Autodesk Fusion 360 part; units mm, degrees
note: some values were not read from the file. Set by a fixed rule: which sketch regions a step uses.
(part 30 of 59)
  spline S54 degree 5 poles (20.9575, -7.61) (20.9576, -7.61) (20.9577, -7.6102) (20.958, -7.6104) (20.9583, -7.6107) (20.9589, -7.6112) (20.9595, -7.6118) (20.9602, -7.6125) (20.961, -7.6132) (20.9619, -7.614) (20.9629, -7.6149) (20.9639, -7.6159) (20.9651, -7.6169) (20.9663, -7.618) (20.9675, -7.6192) (20.9689, -7.6204) (20.9704, -7.6217) (20.9719, -7.623) (20.9735, -7.6245) (20.9752, -7.626) (20.9769, -7.6275) (20.9787, -7.6291) (20.9806, -7.6308) (20.9826, -7.6325) (20.9847, -7.6343) (20.9868, -7.6361) (20.989, -7.638) (20.9912, -7.6399) (20.9936, -7.6419) (20.996, -7.644) (20.9984, -7.6461) (21.001, -7.6482) (21.0036, -7.6504) (21.0063, -7.6527) (21.009, -7.655) (21.0119, -7.6573) (21.0148, -7.6597) (21.0177, -7.6622) (21.0207, -7.6647) (21.0238, -7.6672) (21.027, -7.6698) (21.0302, -7.6724) (21.0335, -7.6751) (21.0368, -7.6778) (21.0403, -7.6806) (21.0437, -7.6834) (21.0473, -7.6862) (21.0509, -7.6891) (21.0546, -7.692) (21.0583, -7.695) (21.0621, -7.698) (21.066, -7.701) (21.0699, -7.7041) (21.0739, -7.7072) (21.0779, -7.7103) (21.082, -7.7135) (21.0862, -7.7167) (21.0904, -7.72) (21.0947, -7.7233) (21.099, -7.7266) (21.1034, -7.73) (21.1079, -7.7333) (21.1124, -7.7368) (21.117, -7.7402) (21.1216, -7.7437) (21.1263, -7.7472) (21.1311, -7.7508) (21.1359, -7.7544) (21.1408, -7.758) (21.1457, -7.7616) (21.1507, -7.7653) (21.1557, -7.769) (21.1608, -7.7727) (21.166, -7.7765) (21.1712, -7.7802) (21.1764, -7.7841) (21.1818, -7.7879) (21.1871, -7.7918) (21.1926, -7.7956) (21.1981, -7.7996) (21.2036, -7.8035) (21.2092, -7.8075) (21.2148, -7.8115) (21.2205, -7.8155) (21.2263, -7.8195) (21.2321, -7.8236) (21.238, -7.8277) (21.2439, -7.8318) (21.2498, -7.8359) (21.2559, -7.8401) (21.2619, -7.8442) (21.2681, -7.8484) (21.2742, -7.8527) (21.2805, -7.8569) (21.2867, -7.8612) (21.2931, -7.8655) (21.2995, -7.8698) (21.3059, -7.8741) (21.3124, -7.8784) (21.3189, -7.8828) (21.3255, -7.8872) (21.3321, -7.8916) (21.3388, -7.896) (21.3455, -7.9004) (21.3523, -7.9049) (21.3592, -7.9094) (21.3661, -7.9139) (21.373, -7.9184) (21.38, -7.9229) (21.387, -7.9274) (21.3941, -7.932) (21.4012, -7.9366) (21.4084, -7.9412) (21.4156, -7.9458) (21.4229, -7.9504) (21.4302, -7.955) (21.4376, -7.9597) (21.445, -7.9644) (21.4525, -7.969) (21.46, -7.9737) (21.4676, -7.9784) (21.4752, -7.9832) (21.4828, -7.9879) (21.4905, -7.9927) (21.4983, -7.9974) (21.5061, -8.0022) (21.5139, -8.007) (21.5218, -8.0118) (21.5297, -8.0166) (21.5377, -8.0214) (21.5458, -8.0263) (21.5538, -8.0311) (21.5619, -8.036) (21.5701, -8.0409) (21.5783, -8.0457) (21.5866, -8.0506) (21.5949, -8.0555) (21.6032, -8.0605) (21.6116, -8.0654) (21.6201, -8.0703) (21.6285, -8.0753) (21.6371, -8.0802) (21.6456, -8.0852) (21.6542, -8.0902) (21.6629, -8.0951) (21.6716, -8.1001) (21.6803, -8.1051) (21.6891, -8.1101) (21.698, -8.1152) (21.7068, -8.1202) (21.7158, -8.1252) (21.7247, -8.1303) (21.7337, -8.1353) (21.7428, -8.1404) (21.7519, -8.1454) (21.761, -8.1505) (21.7702, -8.1556) (21.7794, -8.1607) (21.7887, -8.1658) (21.798, -8.1709) (21.8073, -8.176) (21.8167, -8.1811) (21.8261, -8.1862) (21.8356, -8.1913) (21.8451, -8.1965) (21.8547, -8.2016) (21.8643, -8.2067) (21.8739, -8.2119) (21.8836, -8.217) (21.8933, -8.2222) (21.9031, -8.2274) (21.9129, -8.2325) (21.9228, -8.2377) (21.9326, -8.2429) (21.9426, -8.248) (21.9525, -8.2532) (21.9625, -8.2584) (21.9726, -8.2636) (21.9827, -8.2688) (21.9928, -8.274) (22.003, -8.2792) (22.0132, -8.2844) (22.0235, -8.2896) (22.0337, -8.2948) (22.0441, -8.3) (22.0544, -8.3052) (22.0649, -8.3105) (22.0753, -8.3157) (22.0858, -8.3209) (22.0963, -8.3261) (22.1069, -8.3313) (22.1175, -8.3366) (22.1281, -8.3418) (22.1388, -8.347) (22.1496, -8.3523) (22.1603, -8.3575) (22.1711, -8.3627) (22.182, -8.368) (22.1928, -8.3732) (22.2038, -8.3784) (22.2147, -8.3837) (22.2257, -8.3889) (22.2367, -8.3942) (22.2478, -8.3994) (22.2589, -8.4046) (22.2701, -8.4099) (22.2812, -8.4151) (22.2925, -8.4204) (22.3037, -8.4256) (22.315, -8.4308) (22.3264, -8.4361) (22.3377, -8.4413) (22.3491, -8.4466) (22.3606, -8.4518) (22.3721, -8.457) (22.3836, -8.4623) (22.3951, -8.4675) (22.4067, -8.4727) (22.4184, -8.478) (22.43, -8.4832) (22.4417, -8.4884) (22.4535, -8.4937) (22.4653, -8.4989) (22.4771, -8.5041) (22.4889, -8.5093) (22.5008, -8.5145) (22.5127, -8.5198) (22.5247, -8.525) (22.5367, -8.5302) (22.5487, -8.5354) (22.5608, -8.5406) (22.5729, -8.5458) (22.585, -8.551) (22.5972, -8.5562) (22.6094, -8.5614) (22.6217, -8.5666) (22.6339, -8.5718) (22.6462, -8.577) (22.6586, -8.5822) (22.671, -8.5873) (22.6834, -8.5925) (22.6934, -8.5967) (22.7009, -8.5998) (22.7059, -8.6018) (22.7084, -8.6029) knots 0 0 0 0 0 0 0.00416667 0.00833333 0.0125 0.01666667 0.02083333 0.025 0.02916667 0.03333333 0.0375 0.04166667 0.04583333 0.05 0.05416667 0.05833333 0.0625 0.06666667 0.07083333 0.075 0.07916667 0.08333333 0.0875 0.09166667 0.09583333 0.1 0.10416667 0.10833333 0.1125 0.11666667 0.12083333 0.125 0.12916667 0.13333333 0.1375 0.14166667 0.14583333 0.15 0.15416667 0.15833333 0.1625 0.16666667 0.17083333 0.175 0.17916667 0.18333333 0.1875 0.19166667 0.19583333 0.2 0.20416667 0.20833333 0.2125 0.21666667 0.22083333 0.225 0.22916667 0.23333333 0.2375 0.24166667 0.24583333 0.25 0.25416667 0.25833333 0.2625 0.26666667 0.27083333 0.275 0.27916667 0.28333333 0.2875 0.29166667 0.29583333 0.3 0.30416667 0.30833333 0.3125 0.31666667 0.32083333 0.325 0.32916667 0.33333333 0.3375 0.34166667 0.34583333 0.35 0.35416667 0.35833333 0.3625 0.36666667 0.37083333 0.375 0.37916667 0.38333333 0.3875 0.39166667 0.39583333 0.4 0.40416667 0.40833333 0.4125 0.41666667 0.42083333 0.425 0.42916667 0.43333333 0.4375 0.44166667 0.44583333 0.45 0.45416667 0.45833333 0.4625 0.46666667 0.47083333 0.475 0.47916667 0.48333333 0.4875 0.49166667 0.49583333 0.5 0.50416667 0.50833333 0.5125 0.51666667 0.52083333 0.525 0.52916667 0.53333333 0.5375 0.54166667 0.54583333 0.55 0.55416667 0.55833333 0.5625 0.56666667 0.57083333 0.575 0.57916667 0.58333333 0.5875 0.59166667 0.59583333 0.6 0.60416667 0.60833333 0.6125 0.61666667 0.62083333 0.625 0.62916667 0.63333333 0.6375 0.64166667 0.64583333 0.65 0.65416667 0.65833333 0.6625 0.66666667 0.67083333 0.675 0.67916667 0.68333333 0.6875 0.69166667 0.69583333 0.7 0.70416667 0.70833333 0.7125 0.71666667 0.72083333 0.725 0.72916667 0.73333333 0.7375 0.74166667 0.74583333 0.75 0.75416667 0.75833333 0.7625 0.76666667 0.77083333 0.775 0.77916667 0.78333333 0.7875 0.79166667 0.79583333 0.8 0.80416667 0.80833333 0.8125 0.81666667 0.82083333 0.825 0.82916667 0.83333333 0.8375 0.84166667 0.84583333 0.85 0.85416667 0.85833333 0.8625 0.86666667 0.87083333 0.875 0.87916667 0.88333333 0.8875 0.89166667 0.89583333 0.9 0.90416667 0.90833333 0.9125 0.91666667 0.92083333 0.925 0.92916667 0.93333333 0.9375 0.94166667 0.94583333 0.95 0.95416667 0.95833333 0.9625 0.96666667 0.97083333 0.975 0.97916667 0.98333333 0.9875 0.99166667 0.99583333 1 1 1 1 1 1
  arc A63 (22.7084, -8.6029) -> (23.3609, -7.8781) centre (0, 12.5) ccw
  spline S55 degree 5 poles (23.3609, -7.8781) (23.3596, -7.8757) (23.3571, -7.871) (23.3532, -7.8639) (23.348, -7.8544) (23.3416, -7.8426) (23.3351, -7.8308) (23.3287, -7.819) (23.3222, -7.8073) (23.3158, -7.7957) (23.3094, -7.784) (23.3029, -7.7724) (23.2965, -7.7609) (23.29, -7.7493) (23.2836, -7.7379) (23.2771, -7.7264) (23.2707, -7.715) (23.2643, -7.7036) (23.2578, -7.6922) (23.2514, -7.6809) (23.245, -7.6697) (23.2385, -7.6584) (23.2321, -7.6472) (23.2257, -7.636) (23.2193, -7.6249) (23.2128, -7.6138) (23.2064, -7.6028) (23.2, -7.5917) (23.1936, -7.5808) (23.1872, -7.5698) (23.1807, -7.5589) (23.1743, -7.548) (23.1679, -7.5372) (23.1615, -7.5264) (23.1551, -7.5156) (23.1487, -7.5049) (23.1423, -7.4942) (23.136, -7.4836) (23.1296, -7.473) (23.1232, -7.4624) (23.1168, -7.4518) (23.1104, -7.4413) (23.1041, -7.4309) (23.0977, -7.4205) (23.0914, -7.4101) (23.085, -7.3997) (23.0786, -7.3894) (23.0723, -7.3791) (23.066, -7.3689) (23.0596, -7.3587) (23.0533, -7.3486) (23.047, -7.3384) (23.0406, -7.3284) (23.0343, -7.3183) (23.028, -7.3083) (23.0217, -7.2984) (23.0154, -7.2884) (23.0091, -7.2785) (23.0029, -7.2687) (22.9966, -7.2589) (22.9903, -7.2491) (22.984, -7.2394) (22.9778, -7.2297) (22.9715, -7.22) (22.9653, -7.2104) (22.9591, -7.2009) (22.9528, -7.1913) (22.9466, -7.1818) (22.9404, -7.1724) (22.9342, -7.163) (22.928, -7.1536) (22.9218, -7.1443) (22.9156, -7.135) (22.9095, -7.1257) (22.9033, -7.1165) (22.8971, -7.1073) (22.891, -7.0982) (22.8849, -7.0891) (22.8787, -7.0801) (22.8726, -7.0711) (22.8665, -7.0621) (22.8604, -7.0532) (22.8543, -7.0443) (22.8483, -7.0354) (22.8422, -7.0266) (22.8361, -7.0179) (22.8301, -7.0091) (22.8241, -7.0005) (22.818, -6.9918) (22.812, -6.9832) (22.806, -6.9747) (22.8, -6.9662) (22.7941, -6.9577) (22.7881, -6.9493) (22.7822, -6.9409) (22.7762, -6.9325) (22.7703, -6.9242) (22.7644, -6.916) (22.7585, -6.9078) (22.7526, -6.8996) (22.7467, -6.8914) (22.7408, -6.8834) (22.735, -6.8753) (22.7292, -6.8673) (22.7233, -6.8593) (22.7175, -6.8514) (22.7118, -6.8436) (22.706, -6.8357) (22.7002, -6.8279) (22.6945, -6.8202) (22.6887, -6.8125) (22.683, -6.8048) (22.6773, -6.7972) (22.6716, -6.7897) (22.666, -6.7821) (22.6603, -6.7747) (22.6547, -6.7672) (22.6491, -6.7598) (22.6435, -6.7525) (22.6379, -6.7452) (22.6323, -6.7379) (22.6268, -6.7307) (22.6212, -6.7236) (22.6157, -6.7165) (22.6102, -6.7094) (22.6048, -6.7024) (22.5993, -6.6954) (22.5939, -6.6884) (22.5884, -6.6815) (22.583, -6.6747) (22.5777, -6.6679) (22.5723, -6.6611) (22.567, -6.6544) (22.5617, -6.6478) (22.5564, -6.6412) (22.5511, -6.6346) (22.5458, -6.6281) (22.5406, -6.6216) (22.5354, -6.6152) (22.5302, -6.6088) (22.525, -6.6025) (22.5199, -6.5962) (22.5148, -6.59) (22.5097, -6.5838) (22.5046, -6.5776) (22.4996, -6.5715) (22.4945, -6.5655) (22.4895, -6.5595) (22.4846, -6.5536) (22.4796, -6.5477) (22.4747, -6.5418) (22.4698, -6.536) (22.4649, -6.5303) (22.4601, -6.5246) (22.4553, -6.5189) (22.4505, -6.5133) (22.4457, -6.5077) (22.441, -6.5022) (22.4363, -6.4968) (22.4316, -6.4914) (22.427, -6.486) (22.4223, -6.4807) (22.4177, -6.4755) (22.4132, -6.4703) (22.4087, -6.4651) (22.4042, -6.46) (22.3997, -6.455) (22.3953, -6.45) (22.3909, -6.4451) (22.3865, -6.4402) (22.3821, -6.4353) (22.3778, -6.4306) (22.3736, -6.4258) (22.3693, -6.4211) (22.3651, -6.4165) (22.3609, -6.4119) (22.3568, -6.4074) (22.3527, -6.403) (22.3486, -6.3986) (22.3446, -6.3942) (22.3406, -6.3899) (22.3367, -6.3856) (22.3328, -6.3814) (22.3289, -6.3773) (22.325, -6.3732) (22.3212, -6.3692) (22.3175, -6.3652) (22.3138, -6.3613) (22.3101, -6.3574) (22.3065, -6.3536) (22.3029, -6.3499) (22.2993, -6.3462) (22.2958, -6.3426) (22.2923, -6.339) (22.2889, -6.3355) (22.2855, -6.332) (22.2822, -6.3286) (22.2789, -6.3252) (22.2757, -6.322) (22.2725, -6.3187) (22.2693, -6.3156) (22.2662, -6.3124) (22.2632, -6.3094) (22.2602, -6.3064) (22.2572, -6.3035) (22.2543, -6.3006) (22.2515, -6.2978) (22.2487, -6.2951) (22.2459, -6.2924) (22.2433, -6.2897) (22.2406, -6.2872) (22.238, -6.2847) (22.2355, -6.2823) (22.2331, -6.2799) (22.2307, -6.2776) (22.2283, -6.2753) (22.226, -6.2732) (22.2238, -6.271) (22.2216, -6.269) (22.2195, -6.267) (22.2175, -6.2651) (22.2155, -6.2632) (22.2136, -6.2615) (22.2117, -6.2597) (22.2099, -6.2581) (22.2082, -6.2565) (22.2066, -6.255) (22.205, -6.2536) (22.2035, -6.2522) (22.202, -6.2509) (22.2007, -6.2497) (22.1994, -6.2485) (22.1982, -6.2474) (22.197, -6.2464) (22.196, -6.2455) (22.195, -6.2446) (22.1941, -6.2438) (22.1933, -6.2431) (22.1925, -6.2424) (22.1919, -6.2419) (22.1913, -6.2414) (22.1909, -6.241) (22.1907, -6.2408) (22.1905, -6.2407) (22.1904, -6.2406) knots -1 -1 -1 -1 -1 -1 -0.99583333 -0.99166667 -0.9875 -0.98333333 -0.97916667 -0.975 -0.97083333 -0.96666667 -0.9625 -0.95833333 -0.95416667 -0.95 -0.94583333 -0.94166667 -0.9375 -0.93333333 -0.92916667 -0.925 -0.92083333 -0.91666667 -0.9125 -0.90833333 -0.90416667 -0.9 -0.89583333 -0.89166667 -0.8875 -0.88333333 -0.87916667 -0.875 -0.87083333 -0.86666667 -0.8625 -0.85833333 -0.85416667 -0.85 -0.84583333 -0.84166667 -0.8375 -0.83333333 -0.82916667 -0.825 -0.82083333 -0.81666667 -0.8125 -0.80833333 -0.80416667 -0.8 -0.79583333 -0.79166667 -0.7875 -0.78333333 -0.77916667 -0.775 -0.77083333 -0.76666667 -0.7625 -0.75833333 -0.75416667 -0.75 -0.74583333 -0.74166667 -0.7375 -0.73333333 -0.72916667 -0.725 -0.72083333 -0.71666667 -0.7125 -0.70833333 -0.70416667 -0.7 -0.69583333 -0.69166667 -0.6875 -0.68333333 -0.67916667 -0.675 -0.67083333 -0.66666667 -0.6625 -0.65833333 -0.65416667 -0.65 -0.64583333 -0.64166667 -0.6375 -0.63333333 -0.62916667 -0.625 -0.62083333 -0.61666667 -0.6125 -0.60833333 -0.60416667 -0.6 -0.59583333 -0.59166667 -0.5875 -0.58333333 -0.57916667 -0.575 -0.57083333 -0.56666667 -0.5625 -0.55833333 -0.55416667 -0.55 -0.54583333 -0.54166667 -0.5375 -0.53333333 -0.52916667 -0.525 -0.52083333 -0.51666667 -0.5125 -0.50833333 -0.50416667 -0.5 -0.49583333 -0.49166667 -0.4875 -0.48333333 -0.47916667 -0.475 -0.47083333 -0.46666667 -0.4625 -0.45833333 -0.45416667 -0.45 -0.44583333 -0.44166667 -0.4375 -0.43333333 -0.42916667 -0.425 -0.42083333 -0.41666667 -0.4125 -0.40833333 -0.40416667 -0.4 -0.39583333 -0.39166667 -0.3875 -0.38333333 -0.37916667 -0.375 -0.37083333 -0.36666667 -0.3625 -0.35833333 -0.35416667 -0.35 -0.34583333 -0.34166667 -0.3375 -0.33333333 -0.32916667 -0.325 -0.32083333 -0.31666667 -0.3125 -0.30833333 -0.30416667 -0.3 -0.29583333 -0.29166667 -0.2875 -0.28333333 -0.27916667 -0.275 -0.27083333 -0.26666667 -0.2625 -0.25833333 -0.25416667 -0.25 -0.24583333 -0.24166667 -0.2375 -0.23333333 -0.22916667 -0.225 -0.22083333 -0.21666667 -0.2125 -0.20833333 -0.20416667 -0.2 -0.19583333 -0.19166667 -0.1875 -0.18333333 -0.17916667 -0.175 -0.17083333 -0.16666667 -0.1625 -0.15833333 -0.15416667 -0.15 -0.14583333 -0.14166667 -0.1375 -0.13333333 -0.12916667 -0.125 -0.12083333 -0.11666667 -0.1125 -0.10833333 -0.10416667 -0.1 -0.09583333 -0.09166667 -0.0875 -0.08333333 -0.07916667 -0.075 -0.07083333 -0.06666667 -0.0625 -0.05833333 -0.05416667 -0.05 -0.04583333 -0.04166667 -0.0375 -0.03333333 -0.02916667 -0.025 -0.02083333 -0.01666667 -0.0125 -0.00833333 -0.00416667 0 0 0 0 0 0
  line L111 (22.1904, -6.2406) -> (22.1898, -6.2401)
  line L112 (22.1898, -6.2401) -> (21.9649, -6.0501)
  arc A64 (21.9649, -6.0501) -> (22.7115, -5.1281) centre (0, 12.5) ccw
  line L113 (22.7115, -5.1281) -> (22.9441, -5.3086)
  line L114 (22.9441, -5.3086) -> (22.9448, -5.3091)
  spline S56 degree 5 poles (22.9448, -5.3091) (22.9448, -5.3092) (22.945, -5.3093) (22.9453, -5.3095) (22.9457, -5.3098) (22.9463, -5.3103) (22.9469, -5.3108) (22.9477, -5.3114) (22.9486, -5.312) (22.9496, -5.3127) (22.9506, -5.3135) (22.9518, -5.3144) (22.953, -5.3153) (22.9543, -5.3162) (22.9557, -5.3172) (22.9572, -5.3183) (22.9588, -5.3195) (22.9604, -5.3207) (22.9622, -5.3219) (22.964, -5.3232) (22.9659, -5.3246) (22.9679, -5.326) (22.9699, -5.3274) (22.9721, -5.3289) (22.9743, -5.3305) (22.9766, -5.3321) (22.979, -5.3337) (22.9814, -5.3354) (22.984, -5.3372) (22.9866, -5.3389) (22.9893, -5.3408) (22.992, -5.3427) (22.9948, -5.3446) (22.9978, -5.3465) (23.0007, -5.3485) (23.0038, -5.3506) (23.0069, -5.3527) (23.0101, -5.3548) (23.0134, -5.357) (23.0167, -5.3592) (23.0201, -5.3614) (23.0236, -5.3637) (23.0271, -5.366) (23.0308, -5.3683) (23.0344, -5.3707) (23.0382, -5.3731) (23.042, -5.3756) (23.0459, -5.3781) (23.0499, -5.3806) (23.0539, -5.3831) (23.058, -5.3857) (23.0621, -5.3883) (23.0664, -5.391) (23.0706, -5.3937) (23.075, -5.3964) (23.0794, -5.3991) (23.0839, -5.4019) (23.0884, -5.4047) (23.093, -5.4075) (23.0977, -5.4103) (23.1024, -5.4132) (23.1072, -5.4161) (23.1121, -5.4191) (23.117, -5.422) (23.122, -5.425) (23.127, -5.428) (23.1321, -5.431) (23.1373, -5.4341) (23.1425, -5.4372) (23.1478, -5.4403) (23.1531, -5.4434) (23.1585, -5.4466) (23.164, -5.4497) (23.1695, -5.4529) (23.1751, -5.4562) (23.1807, -5.4594) (23.1864, -5.4627) (23.1921, -5.4659) (23.1979, -5.4692) (23.2038, -5.4726) (23.2097, -5.4759) (23.2157, -5.4793) (23.2217, -5.4826) (23.2278, -5.486) (23.234, -5.4895) (23.2402, -5.4929) (23.2464, -5.4963) (23.2527, -5.4998) (23.2591, -5.5033) (23.2655, -5.5068) (23.272, -5.5103) (23.2785, -5.5139) (23.2851, -5.5174) (23.2918, -5.521) (23.2984, -5.5246) (23.3052, -5.5282) (23.312, -5.5318) (23.3188, -5.5354) (23.3257, -5.539) (23.3327, -5.5427) (23.3397, -5.5464) (23.3468, -5.5501) (23.3539, -5.5538) (23.361, -5.5575) (23.3683, -5.5612) (23.3755, -5.5649) (23.3828, -5.5687) (23.3902, -5.5724) (23.3976, -5.5762) (23.4051, -5.58) (23.4126, -5.5838) (23.4202, -5.5876) (23.4278, -5.5914) (23.4355, -5.5952) (23.4432, -5.5991) (23.451, -5.6029) (23.4588, -5.6068) (23.4666, -5.6106) (23.4746, -5.6145) (23.4825, -5.6184) (23.4905, -5.6223) (23.4986, -5.6262) (23.5067, -5.6301) (23.5149, -5.634) (23.5231, -5.6379) (23.5313, -5.6419) (23.5396, -5.6458) (23.548, -5.6498) (23.5564, -5.6537) (23.5648, -5.6577) (23.5733, -5.6617) (23.5818, -5.6657) (23.5904, -5.6696) (23.5991, -5.6736) (23.6077, -5.6776) (23.6165, -5.6816) (23.6252, -5.6857) (23.634, -5.6897) (23.6429, -5.6937) (23.6518, -5.6977) (23.6607, -5.7018) (23.6697, -5.7058) (23.6788, -5.7098) (23.6879, -5.7139) (23.697, -5.7179) (23.7062, -5.722) (23.7154, -5.726) (23.7247, -5.7301) (23.734, -5.7342) (23.7433, -5.7383) (23.7527, -5.7423) (23.7622, -5.7464) (23.7716, -5.7505) (23.7812, -5.7546) (23.7907, -5.7587) (23.8004, -5.7627) (23.81, -5.7668) (23.8197, -5.7709) (23.8295, -5.775) (23.8393, -5.7791) (23.8491, -5.7832) (23.859, -5.7873) (23.8689, -5.7914) (23.8788, -5.7955) (23.8888, -5.7996) (23.8989, -5.8038) (23.909, -5.8079) (23.9191, -5.812) (23.9292, -5.8161) (23.9395, -5.8202) (23.9497, -5.8243) (23.96, -5.8284) (23.9703, -5.8325) (23.9807, -5.8366) (23.9911, -5.8408) (24.0016, -5.8449) (24.0121, -5.849) (24.0226, -5.8531) (24.0332, -5.8572) (24.0438, -5.8613) (24.0545, -5.8654) (24.0652, -5.8695) (24.0759, -5.8736) (24.0867, -5.8777) (24.0975, -5.8818) (24.1084, -5.8859) (24.1193, -5.89) (24.1302, -5.8941) (24.1412, -5.8982) (24.1522, -5.9023) (24.1633, -5.9064) (24.1744, -5.9105) (24.1855, -5.9146) (24.1967, -5.9187) (24.2079, -5.9228) (24.2191, -5.9269) (24.2304, -5.9309) (24.2417, -5.935) (24.2531, -5.9391) (24.2645, -5.9431) (24.276, -5.9472) (24.2874, -5.9513) (24.299, -5.9553) (24.3105, -5.9594) (24.3221, -5.9634) (24.3337, -5.9675) (24.3454, -5.9715) (24.3571, -5.9756) (24.3689, -5.9796) (24.3806, -5.9836) (24.3925, -5.9877) (24.4043, -5.9917) (24.4162, -5.9957) (24.4281, -5.9997) (24.4401, -6.0037) (24.4521, -6.0077) (24.4642, -6.0117) (24.4762, -6.0157) (24.4884, -6.0197) (24.5005, -6.0237) (24.5127, -6.0277) (24.5249, -6.0316) (24.5372, -6.0356) (24.5495, -6.0395) (24.5618, -6.0435) (24.5742, -6.0475) (24.5866, -6.0514) (24.599, -6.0553) (24.6115, -6.0593) (24.624, -6.0632) (24.6365, -6.0671) (24.6491, -6.071) (24.6617, -6.0749) (24.6744, -6.0788) (24.6871, -6.0827) (24.6998, -6.0866) (24.7125, -6.0905) (24.7253, -6.0943) (24.7382, -6.0982) (24.751, -6.1021) (24.7639, -6.1059) (24.7743, -6.109) (24.782, -6.1113) (24.7872, -6.1128) (24.7898, -6.1136) knots 0 0 0 0 0 0 0.00416667 0.00833333 0.0125 0.01666667 0.02083333 0.025 0.02916667 0.03333333 0.0375 0.04166667 0.04583333 0.05 0.05416667 0.05833333 0.0625 0.06666667 0.07083333 0.075 0.07916667 0.08333333 0.0875 0.09166667 0.09583333 0.1 0.10416667 0.10833333 0.1125 0.11666667 0.12083333 0.125 0.12916667 0.13333333 0.1375 0.14166667 0.14583333 0.15 0.15416667 0.15833333 0.1625 0.16666667 0.17083333 0.175 0.17916667 0.18333333 0.1875 0.19166667 0.19583333 0.2 0.20416667 0.20833333 0.2125 0.21666667 0.22083333 0.225 0.22916667 0.23333333 0.2375 0.24166667 0.24583333 0.25 0.25416667 0.25833333 0.2625 0.26666667 0.27083333 0.275 0.27916667 0.28333333 0.2875 0.29166667 0.29583333 0.3 0.30416667 0.30833333 0.3125 0.31666667 0.32083333 0.325 0.32916667 0.33333333 0.3375 0.34166667 0.34583333 0.35 0.35416667 0.35833333 0.3625 0.36666667 0.37083333 0.375 0.37916667 0.38333333 0.3875 0.39166667 0.39583333 0.4 0.40416667 0.40833333 0.4125 0.41666667 0.42083333 0.425 0.42916667 0.43333333 0.4375 0.44166667 0.44583333 0.45 0.45416667 0.45833333 0.4625 0.46666667 0.47083333 0.475 0.47916667 0.48333333 0.4875 0.49166667 0.49583333 0.5 0.50416667 0.50833333 0.5125 0.51666667 0.52083333 0.525 0.52916667 0.53333333 0.5375 0.54166667 0.54583333 0.55 0.55416667 0.55833333 0.5625 0.56666667 0.57083333 0.575 0.57916667 0.58333333 0.5875 0.59166667 0.59583333 0.6 0.60416667 0.60833333 0.6125 0.61666667 0.62083333 0.625 0.62916667 0.63333333 0.6375 0.64166667 0.64583333 0.65 0.65416667 0.65833333 0.6625 0.66666667 0.67083333 0.675 0.67916667 0.68333333 0.6875 0.69166667 0.69583333 0.7 0.70416667 0.70833333 0.7125 0.71666667 0.72083333 0.725 0.72916667 0.73333333 0.7375 0.74166667 0.74583333 0.75 0.75416667 0.75833333 0.7625 0.76666667 0.77083333 0.775 0.77916667 0.78333333 0.7875 0.79166667 0.79583333 0.8 0.80416667 0.80833333 0.8125 0.81666667 0.82083333 0.825 0.82916667 0.83333333 0.8375 0.84166667 0.84583333 0.85 0.85416667 0.85833333 0.8625 0.86666667 0.87083333 0.875 0.87916667 0.88333333 0.8875 0.89166667 0.89583333 0.9 0.90416667 0.90833333 0.9125 0.91666667 0.92083333 0.925 0.92916667 0.93333333 0.9375 0.94166667 0.94583333 0.95 0.95416667 0.95833333 0.9625 0.96666667 0.97083333 0.975 0.97916667 0.98333333 0.9875 0.99166667 0.99583333 1 1 1 1 1 1
  arc A65 (24.7898, -6.1136) -> (25.363, -5.3246) centre (0, 12.5) ccw
  spline S57 degree 5 poles (25.363, -5.3246) (25.3615, -5.3224) (25.3584, -5.3179) (25.3539, -5.3112) (25.3477, -5.3023) (25.3401, -5.2913) (25.3325, -5.2802) (25.3248, -5.2692) (25.3172, -5.2583) (25.3096, -5.2473) (25.3019, -5.2364) (25.2943, -5.2256) (25.2867, -5.2147) (25.2791, -5.2039) (25.2715, -5.1932) (25.2639, -5.1825) (25.2563, -5.1718) (25.2487, -5.1611) (25.2411, -5.1505) (25.2335, -5.1399) (25.2259, -5.1294) (25.2184, -5.1189) (25.2108, -5.1084) (25.2032, -5.098) (25.1957, -5.0876) (25.1881, -5.0772) (25.1806, -5.0669) (25.1731, -5.0566) (25.1655, -5.0464) (25.158, -5.0361) (25.1505, -5.026) (25.143, -5.0158) (25.1355, -5.0057) (25.128, -4.9956) (25.1205, -4.9856) (25.113, -4.9756) (25.1055, -4.9657) (25.0981, -4.9557) (25.0906, -4.9458) (25.0832, -4.936) (25.0757, -4.9262) (25.0683, -4.9164) (25.0609, -4.9067) (25.0534, -4.897) (25.046, -4.8873) (25.0386, -4.8777) (25.0312, -4.8681) (25.0238, -4.8585) (25.0165, -4.849) (25.0091, -4.8395) (25.0017, -4.8301) (24.9944, -4.8207) (24.9871, -4.8113) (24.9797, -4.802) (24.9724, -4.7927) (24.9651, -4.7835) (24.9578, -4.7743) (24.9505, -4.7651) (24.9432, -4.7559) (24.936, -4.7469) (24.9287, -4.7378) (24.9215, -4.7288) (24.9142, -4.7198) (24.907, -4.7108) (24.8998, -4.7019) (24.8926, -4.6931) (24.8854, -4.6842) (24.8782, -4.6754) (24.8711, -4.6667) (24.8639, -4.658) (24.8568, -4.6493) (24.8496, -4.6407) (24.8425, -4.6321) (24.8354, -4.6235) (24.8283, -4.615) (24.8212, -4.6065) (24.8142, -4.5981) (24.8071, -4.5897) (24.8001, -4.5813) (24.7931, -4.573) (24.7861, -4.5647) (24.7791, -4.5565) (24.7721, -4.5483) (24.7651, -4.5401) (24.7582, -4.532) (24.7512, -4.5239) (24.7443, -4.5159) (24.7374, -4.5079) (24.7305, -4.4999) (24.7236, -4.492) (24.7168, -4.4841) (24.7099, -4.4763) (24.7031, -4.4685) (24.6963, -4.4607) (24.6895, -4.453) (24.6827, -4.4453) (24.6759, -4.4377) (24.6692, -4.4301) (24.6625, -4.4225) (24.6558, -4.415) (24.6491, -4.4075) (24.6424, -4.4001) (24.6357, -4.3927) (24.6291, -4.3854) (24.6225, -4.3781) (24.6159, -4.3708) (24.6093, -4.3636) (24.6027, -4.3564) (24.5962, -4.3492) (24.5897, -4.3421) (24.5831, -4.3351) (24.5767, -4.3281) (24.5702, -4.3211) (24.5638, -4.3142) (24.5573, -4.3073) (24.5509, -4.3004) (24.5446, -4.2936) (24.5382, -4.2869) (24.5319, -4.2801) (24.5255, -4.2735) (24.5192, -4.2668) (24.513, -4.2602) (24.5067, -4.2537) (24.5005, -4.2472) (24.4943, -4.2407) (24.4881, -4.2343) (24.482, -4.2279) (24.4758, -4.2216) (24.4697, -4.2153) (24.4636, -4.2091) (24.4576, -4.2029) (24.4515, -4.1967) (24.4455, -4.1906) (24.4395, -4.1845) (24.4336, -4.1785) (24.4277, -4.1725) (24.4218, -4.1666) (24.4159, -4.1607) (24.41, -4.1549) (24.4042, -4.1491) (24.3984, -4.1433) (24.3926, -4.1376) (24.3869, -4.1319) (24.3812, -4.1263) (24.3755, -4.1207) (24.3698, -4.1152) (24.3642, -4.1097) (24.3586, -4.1043) (24.353, -4.0989) (24.3475, -4.0935) (24.342, -4.0882) (24.3365, -4.083) (24.3311, -4.0778) (24.3257, -4.0726) (24.3203, -4.0675) (24.3149, -4.0624) (24.3096, -4.0574) (24.3043, -4.0524) (24.2991, -4.0475) (24.2939, -4.0426) (24.2887, -4.0378) (24.2835, -4.033) (24.2784, -4.0282) (24.2733, -4.0236) (24.2683, -4.0189) (24.2633, -4.0143) (24.2583, -4.0098) (24.2534, -4.0053) (24.2485, -4.0008) (24.2436, -3.9964) (24.2388, -3.992) (24.234, -3.9877) (24.2293, -3.9835) (24.2246, -3.9793) (24.2199, -3.9751) (24.2153, -3.971) (24.2107, -3.9669) (24.2062, -3.9629) (24.2017, -3.959) (24.1972, -3.955) (24.1928, -3.9512) (24.1884, -3.9474) (24.1841, -3.9436) (24.1798, -3.9399) (24.1755, -3.9362) (24.1713, -3.9326) (24.1672, -3.9291) (24.1631, -3.9256) (24.159, -3.9221) (24.155, -3.9187) (24.151, -3.9153) (24.1471, -3.912) (24.1432, -3.9088) (24.1394, -3.9056) (24.1356, -3.9024) (24.1319, -3.8994) (24.1283, -3.8963) (24.1246, -3.8933) (24.1211, -3.8904) (24.1176, -3.8875) (24.1141, -3.8847) (24.1107, -3.8819) (24.1073, -3.8792) (24.104, -3.8766) (24.1008, -3.874) (24.0976, -3.8714) (24.0945, -3.8689) (24.0914, -3.8665) (24.0884, -3.8641) (24.0855, -3.8618) (24.0826, -3.8595) (24.0798, -3.8573) (24.077, -3.8551) (24.0743, -3.853) (24.0717, -3.851) (24.0691, -3.849) (24.0666, -3.8471) (24.0641, -3.8452) (24.0618, -3.8434) (24.0595, -3.8416) (24.0572, -3.8399) (24.0551, -3.8383) (24.053, -3.8367) (24.051, -3.8352) (24.049, -3.8338) (24.0471, -3.8324) (24.0453, -3.831) (24.0436, -3.8298) (24.042, -3.8286) (24.0404, -3.8274) (24.0389, -3.8263) (24.0375, -3.8253) (24.0362, -3.8244) (24.035, -3.8235) (24.0338, -3.8227) (24.0327, -3.8219) (24.0317, -3.8212) (24.0309, -3.8206) (24.0301, -3.82) (24.0294, -3.8195) (24.0287, -3.8191) (24.0283, -3.8188) (24.0281, -3.8186) (24.0279, -3.8185) (24.0278, -3.8184) knots -1 -1 -1 -1 -1 -1 -0.99583333 -0.99166667 -0.9875 -0.98333333 -0.97916667 -0.975 -0.97083333 -0.96666667 -0.9625 -0.95833333 -0.95416667 -0.95 -0.94583333 -0.94166667 -0.9375 -0.93333333 -0.92916667 -0.925 -0.92083333 -0.91666667 -0.9125 -0.90833333 -0.90416667 -0.9 -0.89583333 -0.89166667 -0.8875 -0.88333333 -0.87916667 -0.875 -0.87083333 -0.86666667 -0.8625 -0.85833333 -0.85416667 -0.85 -0.84583333 -0.84166667 -0.8375 -0.83333333 -0.82916667 -0.825 -0.82083333 -0.81666667 -0.8125 -0.80833333 -0.80416667 -0.8 -0.79583333 -0.79166667 -0.7875 -0.78333333 -0.77916667 -0.775 -0.77083333 -0.76666667 -0.7625 -0.75833333 -0.75416667 -0.75 -0.74583333 -0.74166667 -0.7375 -0.73333333 -0.72916667 -0.725 -0.72083333 -0.71666667 -0.7125 -0.70833333 -0.70416667 -0.7 -0.69583333 -0.69166667 -0.6875 -0.68333333 -0.67916667 -0.675 -0.67083333 -0.66666667 -0.6625 -0.65833333 -0.65416667 -0.65 -0.64583333 -0.64166667 -0.6375 -0.63333333 -0.62916667 -0.625 -0.62083333 -0.61666667 -0.6125 -0.60833333 -0.60416667 -0.6 -0.59583333 -0.59166667 -0.5875 -0.58333333 -0.57916667 -0.575 -0.57083333 -0.56666667 -0.5625 -0.55833333 -0.55416667 -0.55 -0.54583333 -0.54166667 -0.5375 -0.53333333 -0.52916667 -0.525 -0.52083333 -0.51666667 -0.5125 -0.50833333 -0.50416667 -0.5 -0.49583333 -0.49166667 -0.4875 -0.48333333 -0.47916667 -0.475 -0.47083333 -0.46666667 -0.4625 -0.45833333 -0.45416667 -0.45 -0.44583333 -0.44166667 -0.4375 -0.43333333 -0.42916667 -0.425 -0.42083333 -0.41666667 -0.4125 -0.40833333 -0.40416667 -0.4 -0.39583333 -0.39166667 -0.3875 -0.38333333 -0.37916667 -0.375 -0.37083333 -0.36666667 -0.3625 -0.35833333 -0.35416667 -0.35 -0.34583333 -0.34166667 -0.3375 -0.33333333 -0.32916667 -0.325 -0.32083333 -0.31666667 -0.3125 -0.30833333 -0.30416667 -0.3 -0.29583333 -0.29166667 -0.2875 -0.28333333 -0.27916667 -0.275 -0.27083333 -0.26666667 -0.2625 -0.25833333 -0.25416667 -0.25 -0.24583333 -0.24166667 -0.2375 -0.23333333 -0.22916667 -0.225 -0.22083333 -0.21666667 -0.2125 -0.20833333 -0.20416667 -0.2 -0.19583333 -0.19166667 -0.1875 -0.18333333 -0.17916667 -0.175 -0.17083333 -0.16666667 -0.1625 -0.15833333 -0.15416667 -0.15 -0.14583333 -0.14166667 -0.1375 -0.13333333 -0.12916667 -0.125 -0.12083333 -0.11666667 -0.1125 -0.10833333 -0.10416667 -0.1 -0.09583333 -0.09166667 -0.0875 -0.08333333 -0.07916667 -0.075 -0.07083333 -0.06666667 -0.0625 -0.05833333 -0.05416667 -0.05 -0.04583333 -0.04166667 -0.0375 -0.03333333 -0.02916667 -0.025 -0.02083333 -0.01666667 -0.0125 -0.00833333 -0.00416667 0 0 0 0 0 0
  line L115 (24.0278, -3.8184) -> (24.0271, -3.818)
  line L116 (24.0271, -3.818) -> (23.7836, -3.6526)
  arc A66 (23.7836, -3.6526) -> (24.4297, -2.6575) centre (0, 12.5) ccw
  line L117 (24.4297, -2.6575) -> (24.6799, -2.8128)
  line L118 (24.6799, -2.8128) -> (24.6806, -2.8132)
  spline S58 degree 5 poles (24.6806, -2.8132) (24.6807, -2.8132) (24.6809, -2.8133) (24.6812, -2.8135) (24.6816, -2.8138) (24.6822, -2.8142) (24.683, -2.8146) (24.6838, -2.8151) (24.6848, -2.8157) (24.6858, -2.8163) (24.6869, -2.8169) (24.6881, -2.8177) (24.6895, -2.8184) (24.6909, -2.8193) (24.6924, -2.8201) (24.694, -2.821) (24.6956, -2.822) (24.6974, -2.823) (24.6993, -2.8241) (24.7012, -2.8252) (24.7033, -2.8263) (24.7054, -2.8275) (24.7076, -2.8287) (24.7099, -2.83) (24.7122, -2.8313) (24.7147, -2.8327) (24.7172, -2.8341) (24.7198, -2.8355) (24.7225, -2.837) (24.7253, -2.8385) (24.7282, -2.84) (24.7311, -2.8416) (24.7341, -2.8432) (24.7372, -2.8449) (24.7404, -2.8465) (24.7437, -2.8482) (24.747, -2.85) (24.7504, -2.8518) (24.7539, -2.8536) (24.7574, -2.8554) (24.761, -2.8573) (24.7647, -2.8592) (24.7685, -2.8611) (24.7723, -2.8631) (24.7763, -2.8651) (24.7802, -2.8671) (24.7843, -2.8691) (24.7884, -2.8712) (24.7926, -2.8733) (24.7969, -2.8754) (24.8012, -2.8775) (24.8056, -2.8797) (24.8101, -2.8819) (24.8147, -2.8841) (24.8193, -2.8863) (24.8239, -2.8886) (24.8287, -2.8909) (24.8335, -2.8932) (24.8384, -2.8955) (24.8433, -2.8979) (24.8483, -2.9002) (24.8534, -2.9026) (24.8585, -2.905) (24.8637, -2.9075) (24.869, -2.9099) (24.8743, -2.9124) (24.8797, -2.9149) (24.8852, -2.9174) (24.8907, -2.9199) (24.8962, -2.9224) (24.9019, -2.925) (24.9076, -2.9275) (24.9133, -2.9301) (24.9192, -2.9327) (24.925, -2.9353) (24.931, -2.938) (24.937, -2.9406) (24.943, -2.9433) (24.9492, -2.946) (24.9553, -2.9486) (24.9616, -2.9514) (24.9679, -2.9541) (24.9742, -2.9568) (24.9806, -2.9595) (24.9871, -2.9623) (24.9936, -2.9651) (25.0002, -2.9678) (25.0069, -2.9706) (25.0136, -2.9734) (25.0203, -2.9762) (25.0271, -2.9791) (25.034, -2.9819) (25.0409, -2.9848) (25.0479, -2.9876) (25.0549, -2.9905) (25.062, -2.9933) (25.0691, -2.9962) (25.0763, -2.9991) (25.0836, -3.002) (25.0909, -3.0049) (25.0982, -3.0078) (25.1056, -3.0108) (25.1131, -3.0137) (25.1206, -3.0166) (25.1282, -3.0196) (25.1358, -3.0226) (25.1434, -3.0255) (25.1512, -3.0285) (25.1589, -3.0315) (25.1668, -3.0344) (25.1746, -3.0374) (25.1826, -3.0404) (25.1905, -3.0434) (25.1986, -3.0464) (25.2066, -3.0494) (25.2148, -3.0524) (25.2229, -3.0555) (25.2312, -3.0585) (25.2394, -3.0615) (25.2478, -3.0645) (25.2562, -3.0676) (25.2646, -3.0706) (25.2731, -3.0737) (25.2816, -3.0767) (25.2901, -3.0798) (25.2988, -3.0828) (25.3074, -3.0859) (25.3161, -3.0889) (25.3249, -3.092) (25.3337, -3.095) (25.3426, -3.0981) (25.3515, -3.1012) (25.3604, -3.1042) (25.3694, -3.1073) (25.3785, -3.1104) (25.3876, -3.1134) (25.3967, -3.1165) (25.4059, -3.1196) (25.4151, -3.1227) (25.4244, -3.1257) (25.4337, -3.1288) (25.4431, -3.1319) (25.4525, -3.135) (25.462, -3.138) (25.4715, -3.1411) (25.481, -3.1442) (25.4906, -3.1473) (25.5003, -3.1503) (25.5099, -3.1534) (25.5197, -3.1565) (25.5294, -3.1596) (25.5393, -3.1626) (25.5491, -3.1657) (25.559, -3.1688) (25.569, -3.1718) (25.579, -3.1749) (25.589, -3.1779) (25.5991, -3.181) (25.6092, -3.1841) (25.6194, -3.1871) (25.6296, -3.1902) (25.6398, -3.1932) (25.6501, -3.1963) (25.6604, -3.1993) (25.6708, -3.2023) (25.6812, -3.2054) (25.6917, -3.2084) (25.7022, -3.2114) (25.7127, -3.2145) (25.7233, -3.2175) (25.7339, -3.2205) (25.7446, -3.2235) (25.7553, -3.2265) (25.766, -3.2295) (25.7768, -3.2325) (25.7877, -3.2355) (25.7985, -3.2385) (25.8094, -3.2415) (25.8204, -3.2445) (25.8314, -3.2475) (25.8424, -3.2504) (25.8535, -3.2534) (25.8646, -3.2564) (25.8757, -3.2593) (25.8869, -3.2623) (25.8982, -3.2652) (25.9094, -3.2682) (25.9207, -3.2711) (25.9321, -3.274) (25.9435, -3.2769) (25.9549, -3.2798) (25.9663, -3.2828) (25.9778, -3.2857) (25.9894, -3.2886) (26.001, -3.2914) (26.0126, -3.2943) (26.0242, -3.2972) (26.0359, -3.3001) (26.0477, -3.3029) (26.0594, -3.3058) (26.0712, -3.3086) (26.0831, -3.3115) (26.095, -3.3143) (26.1069, -3.3171) (26.1188, -3.3199) (26.1308, -3.3227) (26.1428, -3.3255) (26.1549, -3.3283) (26.167, -3.3311) (26.1792, -3.3339) (26.1913, -3.3367) (26.2035, -3.3394) (26.2158, -3.3422) (26.2281, -3.3449) (26.2404, -3.3477) (26.2528, -3.3504) (26.2651, -3.3531) (26.2776, -3.3558) (26.29, -3.3585) (26.3025, -3.3612) (26.3151, -3.3639) (26.3276, -3.3666) (26.3403, -3.3692) (26.3529, -3.3719) (26.3656, -3.3745) (26.3783, -3.3771) (26.391, -3.3798) (26.4038, -3.3824) (26.4166, -3.385) (26.4295, -3.3876) (26.4424, -3.3902) (26.4553, -3.3927) (26.4682, -3.3953) (26.4812, -3.3979) (26.4943, -3.4004) (26.5073, -3.4029) (26.5204, -3.4055) (26.5335, -3.408) (26.5467, -3.4105) (26.5599, -3.413) (26.5731, -3.4154) (26.5837, -3.4174) (26.5917, -3.4189) (26.597, -3.4199) (26.5997, -3.4204) knots 0 0 0 0 0 0 0.00416667 0.00833333 0.0125 0.01666667 0.02083333 0.025 0.02916667 0.03333333 0.0375 0.04166667 0.04583333 0.05 0.05416667 0.05833333 0.0625 0.06666667 0.07083333 0.075 0.07916667 0.08333333 0.0875 0.09166667 0.09583333 0.1 0.10416667 0.10833333 0.1125 0.11666667 0.12083333 0.125 0.12916667 0.13333333 0.1375 0.14166667 0.14583333 0.15 0.15416667 0.15833333 0.1625 0.16666667 0.17083333 0.175 0.17916667 0.18333333 0.1875 0.19166667 0.19583333 0.2 0.20416667 0.20833333 0.2125 0.21666667 0.22083333 0.225 0.22916667 0.23333333 0.2375 0.24166667 0.24583333 0.25 0.25416667 0.25833333 0.2625 0.26666667 0.27083333 0.275 0.27916667 0.28333333 0.2875 0.29166667 0.29583333 0.3 0.30416667 0.30833333 0.3125 0.31666667 0.32083333 0.325 0.32916667 0.33333333 0.3375 0.34166667 0.34583333 0.35 0.35416667 0.35833333 0.3625 0.36666667 0.37083333 0.375 0.37916667 0.38333333 0.3875 0.39166667 0.39583333 0.4 0.40416667 0.40833333 0.4125 0.41666667 0.42083333 0.425 0.42916667 0.43333333 0.4375 0.44166667 0.44583333 0.45 0.45416667 0.45833333 0.4625 0.46666667 0.47083333 0.475 0.47916667 0.48333333 0.4875 0.49166667 0.49583333 0.5 0.50416667 0.50833333 0.5125 0.51666667 0.52083333 0.525 0.52916667 0.53333333 0.5375 0.54166667 0.54583333 0.55 0.55416667 0.55833333 0.5625 0.56666667 0.57083333 0.575 0.57916667 0.58333333 0.5875 0.59166667 0.59583333 0.6 0.60416667 0.60833333 0.6125 0.61666667 0.62083333 0.625 0.62916667 0.63333333 0.6375 0.64166667 0.64583333 0.65 0.65416667 0.65833333 0.6625 0.66666667 0.67083333 0.675 0.67916667 0.68333333 0.6875 0.69166667 0.69583333 0.7 0.70416667 0.70833333 0.7125 0.71666667 0.72083333 0.725 0.72916667 0.73333333 0.7375 0.74166667 0.74583333 0.75 0.75416667 0.75833333 0.7625 0.76666667 0.77083333 0.775 0.77916667 0.78333333 0.7875 0.79166667 0.79583333 0.8 0.80416667 0.80833333 0.8125 0.81666667 0.82083333 0.825 0.82916667 0.83333333 0.8375 0.84166667 0.84583333 0.85 0.85416667 0.85833333 0.8625 0.86666667 0.87083333 0.875 0.87916667 0.88333333 0.8875 0.89166667 0.89583333 0.9 0.90416667 0.90833333 0.9125 0.91666667 0.92083333 0.925 0.92916667 0.93333333 0.9375 0.94166667 0.94583333 0.95 0.95416667 0.95833333 0.9625 0.96666667 0.97083333 0.975 0.97916667 0.98333333 0.9875 0.99166667 0.99583333 1 1 1 1 1 1
  arc A67 (26.5997, -3.4204) -> (27.0873, -2.5758) centre (0, 12.5) ccw
  spline S59 degree 5 poles (27.0873, -2.5758) (27.0855, -2.5737) (27.082, -2.5696) (27.0767, -2.5635) (27.0697, -2.5553) (27.061, -2.545) (27.0522, -2.5349) (27.0435, -2.5247) (27.0347, -2.5146) (27.026, -2.5045) (27.0173, -2.4945) (27.0086, -2.4845) (26.9999, -2.4745) (26.9912, -2.4646) (26.9825, -2.4547) (26.9738, -2.4448) (26.9651, -2.435) (26.9565, -2.4252) (26.9478, -2.4154) (26.9392, -2.4057) (26.9305, -2.396) (26.9219, -2.3863) (26.9133, -2.3767) (26.9047, -2.3671) (26.8961, -2.3576) (26.8875, -2.3481) (26.8789, -2.3386) (26.8703, -2.3291) (26.8618, -2.3197) (26.8532, -2.3104) (26.8447, -2.301) (26.8361, -2.2917) (26.8276, -2.2824) (26.8191, -2.2732) (26.8106, -2.264) (26.8021, -2.2549) (26.7937, -2.2457) (26.7852, -2.2366) (26.7767, -2.2276) (26.7683, -2.2186) (26.7599, -2.2096) (26.7515, -2.2006) (26.7431, -2.1917) (26.7347, -2.1829) (26.7263, -2.174) (26.7179, -2.1652) (26.7096, -2.1565) (26.7012, -2.1477) (26.6929, -2.139) (26.6846, -2.1304) (26.6763, -2.1218) (26.668, -2.1132) (26.6597, -2.1046) (26.6514, -2.0961) (26.6432, -2.0877) (26.635, -2.0792) (26.6267, -2.0708) (26.6185, -2.0625) (26.6103, -2.0541) (26.6022, -2.0459) (26.594, -2.0376) (26.5858, -2.0294) (26.5777, -2.0212) (26.5696, -2.0131) (26.5615, -2.005) (26.5534, -1.9969) (26.5453, -1.9889) (26.5373, -1.9809) (26.5292, -1.9729) (26.5212, -1.965) (26.5132, -1.9571) (26.5052, -1.9493) (26.4972, -1.9415) (26.4893, -1.9337) (26.4813, -1.926) (26.4734, -1.9183) (26.4655, -1.9106) (26.4576, -1.903) (26.4497, -1.8954) (26.4419, -1.8879) (26.434, -1.8804) (26.4262, -1.8729) (26.4184, -1.8655) (26.4106, -1.8581) (26.4029, -1.8508) (26.3951, -1.8435) (26.3874, -1.8362) (26.3797, -1.8289) (26.372, -1.8217) (26.3643, -1.8146) (26.3567, -1.8075) (26.3491, -1.8004) (26.3414, -1.7933) (26.3339, -1.7863) (26.3263, -1.7794) (26.3188, -1.7724) (26.3112, -1.7656) (26.3037, -1.7587) (26.2962, -1.7519) (26.2888, -1.7451) (26.2813, -1.7384) (26.2739, -1.7317) (26.2665, -1.725) (26.2592, -1.7184) (26.2518, -1.7119) (26.2445, -1.7053) (26.2372, -1.6988) (26.2299, -1.6924) (26.2227, -1.6859) (26.2154, -1.6796) (26.2082, -1.6732) (26.201, -1.6669) (26.1939, -1.6607) (26.1868, -1.6544) (26.1796, -1.6483) (26.1726, -1.6421) (26.1655, -1.636) (26.1585, -1.63) (26.1515, -1.6239) (26.1445, -1.618) (26.1375, -1.612) (26.1306, -1.6061) (26.1237, -1.6003) (26.1168, -1.5945) (26.11, -1.5887) (26.1032, -1.5829) (26.0964, -1.5772) (26.0896, -1.5716) (26.0829, -1.566) (26.0762, -1.5604) (26.0695, -1.5549) (26.0629, -1.5494) (26.0563, -1.5439) (26.0497, -1.5385) (26.0431, -1.5332) (26.0366, -1.5278) (26.0301, -1.5225) (26.0236, -1.5173) (26.0172, -1.5121) (26.0108, -1.5069) (26.0044, -1.5018) (25.9981, -1.4967) (25.9918, -1.4917) (25.9855, -1.4867) (25.9793, -1.4818) (25.9731, -1.4769) (25.9669, -1.472) (25.9608, -1.4672) (25.9547, -1.4624) (25.9486, -1.4576) (25.9426, -1.4529) (25.9366, -1.4483) (25.9306, -1.4437) (25.9247, -1.4391) (25.9188, -1.4346) (25.913, -1.4301) (25.9072, -1.4257) (25.9014, -1.4213) (25.8957, -1.4169) (25.89, -1.4126) (25.8843, -1.4083) (25.8787, -1.4041) (25.8731, -1.3999) (25.8676, -1.3958) (25.8621, -1.3917) (25.8566, -1.3876) (25.8512, -1.3836) (25.8458, -1.3797) (25.8405, -1.3758) (25.8352, -1.3719) (25.8299, -1.3681) (25.8247, -1.3643) (25.8195, -1.3605) (25.8144, -1.3568) (25.8093, -1.3532) (25.8043, -1.3496) (25.7993, -1.346) (25.7944, -1.3425) (25.7895, -1.339) (25.7847, -1.3356) (25.7799, -1.3322) (25.7751, -1.3289) (25.7704, -1.3256) (25.7658, -1.3224) (25.7612, -1.3192) (25.7566, -1.316) (25.7521, -1.3129) (25.7476, -1.3098) (25.7432, -1.3068) (25.7389, -1.3039) (25.7346, -1.3009) (25.7304, -1.2981) (25.7262, -1.2952) (25.722, -1.2925) (25.718, -1.2897) (25.7139, -1.287) (25.71, -1.2844) (25.706, -1.2818) (25.7022, -1.2793) (25.6984, -1.2768) (25.6947, -1.2743) (25.691, -1.2719) (25.6874, -1.2696) (25.6838, -1.2673) (25.6803, -1.265) (25.6769, -1.2628) (25.6735, -1.2607) (25.6702, -1.2586) (25.667, -1.2565) (25.6638, -1.2545) (25.6607, -1.2526) (25.6577, -1.2506) (25.6547, -1.2488) (25.6518, -1.247) (25.6489, -1.2452) (25.6462, -1.2435) (25.6435, -1.2419) (25.6409, -1.2403) (25.6383, -1.2387) (25.6358, -1.2372) (25.6334, -1.2358) (25.6311, -1.2344) (25.6289, -1.233) (25.6267, -1.2317) (25.6246, -1.2305) (25.6226, -1.2293) (25.6207, -1.2282) (25.6188, -1.2271) (25.6171, -1.2261) (25.6154, -1.2251) (25.6138, -1.2242) (25.6123, -1.2233) (25.6109, -1.2225) (25.6096, -1.2217) (25.6083, -1.221) (25.6072, -1.2204) (25.6061, -1.2198) (25.6052, -1.2193) (25.6043, -1.2188) (25.6036, -1.2184) (25.6029, -1.218) (25.6025, -1.2178) (25.6022, -1.2176) (25.602, -1.2175) (25.6019, -1.2175) knots -1 -1 -1 -1 -1 -1 -0.99583333 -0.99166667 -0.9875 -0.98333333 -0.97916667 -0.975 -0.97083333 -0.96666667 -0.9625 -0.95833333 -0.95416667 -0.95 -0.94583333 -0.94166667 -0.9375 -0.93333333 -0.92916667 -0.925 -0.92083333 -0.91666667 -0.9125 -0.90833333 -0.90416667 -0.9 -0.89583333 -0.89166667 -0.8875 -0.88333333 -0.87916667 -0.875 -0.87083333 -0.86666667 -0.8625 -0.85833333 -0.85416667 -0.85 -0.84583333 -0.84166667 -0.8375 -0.83333333 -0.82916667 -0.825 -0.82083333 -0.81666667 -0.8125 -0.80833333 -0.80416667 -0.8 -0.79583333 -0.79166667 -0.7875 -0.78333333 -0.77916667 -0.775 -0.77083333 -0.76666667 -0.7625 -0.75833333 -0.75416667 -0.75 -0.74583333 -0.74166667 -0.7375 -0.73333333 -0.72916667 -0.725 -0.72083333 -0.71666667 -0.7125 -0.70833333 -0.70416667 -0.7 -0.69583333 -0.69166667 -0.6875 -0.68333333 -0.67916667 -0.675 -0.67083333 -0.66666667 -0.6625 -0.65833333 -0.65416667 -0.65 -0.64583333 -0.64166667 -0.6375 -0.63333333 -0.62916667 -0.625 -0.62083333 -0.61666667 -0.6125 -0.60833333 -0.60416667 -0.6 -0.59583333 -0.59166667 -0.5875 -0.58333333 -0.57916667 -0.575 -0.57083333 -0.56666667 -0.5625 -0.55833333 -0.55416667 -0.55 -0.54583333 -0.54166667 -0.5375 -0.53333333 -0.52916667 -0.525 -0.52083333 -0.51666667 -0.5125 -0.50833333 -0.50416667 -0.5 -0.49583333 -0.49166667 -0.4875 -0.48333333 -0.47916667 -0.475 -0.47083333 -0.46666667 -0.4625 -0.45833333 -0.45416667 -0.45 -0.44583333 -0.44166667 -0.4375 -0.43333333 -0.42916667 -0.425 -0.42083333 -0.41666667 -0.4125 -0.40833333 -0.40416667 -0.4 -0.39583333 -0.39166667 -0.3875 -0.38333333 -0.37916667 -0.375 -0.37083333 -0.36666667 -0.3625 -0.35833333 -0.35416667 -0.35 -0.34583333 -0.34166667 -0.3375 -0.33333333 -0.32916667 -0.325 -0.32083333 -0.31666667 -0.3125 -0.30833333 -0.30416667 -0.3 -0.29583333 -0.29166667 -0.2875 -0.28333333 -0.27916667 -0.275 -0.27083333 -0.26666667 -0.2625 -0.25833333 -0.25416667 -0.25 -0.24583333 -0.24166667 -0.2375 -0.23333333 -0.22916667 -0.225 -0.22083333 -0.21666667 -0.2125 -0.20833333 -0.20416667 -0.2 -0.19583333 -0.19166667 -0.1875 -0.18333333 -0.17916667 -0.175 -0.17083333 -0.16666667 -0.1625 -0.15833333 -0.15416667 -0.15 -0.14583333 -0.14166667 -0.1375 -0.13333333 -0.12916667 -0.125 -0.12083333 -0.11666667 -0.1125 -0.10833333 -0.10416667 -0.1 -0.09583333 -0.09166667 -0.0875 -0.08333333 -0.07916667 -0.075 -0.07083333 -0.06666667 -0.0625 -0.05833333 -0.05416667 -0.05 -0.04583333 -0.04166667 -0.0375 -0.03333333 -0.02916667 -0.025 -0.02083333 -0.01666667 -0.0125 -0.00833333 -0.00416667 0 0 0 0 0 0
  line L119 (25.6019, -1.2175) -> (25.6012, -1.2171)
  line L120 (25.6012, -1.2171) -> (25.3417, -1.078)
  arc A68 (25.3417, -1.078) -> (25.8803, -0.0209) centre (0, 12.5) ccw
  line L121 (25.8803, -0.0209) -> (26.1453, -0.1491)
  line L122 (26.1453, -0.1491) -> (26.1461, -0.1495)